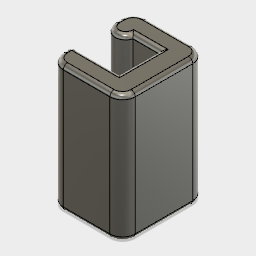
BedClamp v3 (Autodesk Fusion 360 design; units mm, degrees)
Autodesk Fusion 360 part; units mm, degrees
note: some values were not read from the file. Chosen so that the rebuilt part matches the saved one: which face or edge a step refers to. Set by a fixed rule: which sketch regions a step uses.
sketch "Sketch1" plane through (0, 0, 0) normal (0, 1, 0) x (1, 0, 0)
  line L0 (0, 0) -> (10, 0)
  line L1 (10, 0) -> (10, 8.8)
  line L2 (10, 8.8) -> (0, 8.8)
  line L3 (0, 0) -> (0, -5)
  line L4 (0, -5) -> (15, -5)
  line L5 (15, -5) -> (15, 0)
  line L6 (15, 0) -> (0, 0)
  line L7 (10, 0) -> (15, 0)
  line L8 (15, 0) -> (15, 13.8)
  line L9 (15, 13.8) -> (10, 13.8)
  line L10 (10, 13.8) -> (10, 0)
  line L11 (10, 13.8) -> (0, 13.8)
  line L12 (0, 13.8) -> (0, 8.8)
  line L13 (0, 8.8) -> (10, 8.8)
  line L14 (10, 8.8) -> (10, 13.8)
  line L15 (2.5, 7) -> (2.5, 9.5)
  circle A0 centre (2.5, 9.5) radius 2.5
  dimension "d1" = 8.8
  dimension "d2" = 13.8
  dimension "d4" = 2.5
  measures "d1" distance of L0.start L2.end
  measures "d2" distance of L0.end L9.end
  measures "d4" distance of L15.start L15.end
extrude "Extrude1" add sketch "Sketch1" along normal blind 30 contours L1 L6 L7 L8 L9 L10 L14 | L2 L10 L11 L12 L13 L14 A0 | L2 L13 L15 A0 | L2 L13 A0 | L2 L13 L15 A0 makes body 1
extrude "Extrude2" add 1 faces at (15, 10, -4.6) along direction (1, 0, 0) blind 10 on bodies 1 bodies 1
sketch "Sketch2" plane through (0, 0, 0) normal (0, 0, 1) x (1, 0, 0)
  line L0 (10, 0) -> (25, 0)
  line L1 (25, 0) -> (25, 30)
  line L2 (25, 30) -> (10, 30)
  line L3 (10, 30) -> (10, 0)
  line L4 (12, 15) -> (-113, 15)
  circle A0 centre (-113, 15) radius 125
  line L5 (17.5, 30) -> (17.5, 0)
  line L6 (17.5, 0) -> (0, 0)
  line L7 (0, 0) -> (0, 30)
  line L8 (0, 30) -> (17.5, 30)
  line L9 (0, 0) -> (0, 30)
  dimension "d9" = 125
  measures "d9" distance of L4.start L4.end
extrude "Extrude3" cut sketch "Sketch2" against normal blind 8.8 contours L0 L3 L4 A0 L6 | L2 L3 L4 A0 L8 bodies 1
sketch "Sketch3" plane through (0, 0, 0) normal (0, 0, 1) x (1, 0, 0)
  arc A0 (11.0967, 0) -> (11.0967, 30) centre (-113, 15) ccw
  line L0 (11.0967, 0) -> (25, 0)
  line L1 (25, 0) -> (25, 30)
  line L2 (25, 30) -> (11.0967, 30)
extrude "Extrude4" cut 1 faces at (25, 10, -4.6) along direction (-1, 0, 0) blind 8 on bodies 1 bodies 1
extrude "Extrude5" add sketch "Sketch2" along normal blind 5 contours L0 L2 A0 L5 L6 L8 | L0 L3 L4 A0 L6 | L3 L4 L6 L7 L9 | L2 L3 L4 A0 L8 | L3 L4 L7 L8 L9 bodies 1
extrude "Extrude6" cut 1 faces at (17.5, 20, 1.6667) along direction (-1, 0, 0) blind 0.5 on bodies 1 bodies 1
fillet "Fillet1" radius 1 1 edges at (0, 15, 0) on bodies 1
fillet "Fillet2" radius 3 4 edges at (17, 15, -13.8) (0, 15, -13.8) (0, 15, 5) (17, 15, 5) on bodies 1
fillet "Fillet3" radius 1 14 edges at (6.0484, 30, 0) (0.2929, 30, 0.2929) (0, 30, 1.5) (0.8787, 30, 4.1213) (8.5, 30, 5) (16.1213, 30, 4.1213) (17, 30, -4.4) (16.1213, 30, -12.9213) (8.5, 30, -13.8) (0.8787, 30, -12.9213) (0, 30, -10.15) (2.1464, 30, -7.0251) (7.9984, 30, -8.8) (11.0967, 30, -4.4) on bodies 1
fillet "Fillet4" radius 1 14 edges at (11.0967, 0, -4.4) (6.0484, 0, 0) (0.2929, 0, 0.2929) (0, 0, 1.5) (0.8787, 0, 4.1213) (8.5, 0, 5) (16.1213, 0, 4.1213) (17, 0, -4.4) (16.1213, 0, -12.9213) (8.5, 0, -13.8) (0.8787, 0, -12.9213) (0, 0, -10.15) (2.1464, 0, -7.0251) (7.9984, 0, -8.8) on bodies 1
ref_plane "WorkPlane1" through (8.5, 15, -3.8) normal (0, 0, -1) x (-1, 0, 0)
split "Split1" by plane through (8.5, 15, -3.8) normal (0, 0, -1) bodies 1 makes body 2 at (10.3333, 10.3333, -13.8)
move_body "Move1" bodies 2 to x (1, 0, 0) y (0, 1, 0) z (0, 0, 1) at (0, 0, -1.5)
extrude "Extrude7" add 1 faces at (15.3046, 16.546, -3.8) along direction (0, 0, -1) blind 0.75 on bodies 1 bodies 1
move_body "Move2" bodies 2 to x (1, 0, 0) y (0, 1, 0) z (0, 0, 1) at (0, 0, 0.75)
combine "Combine1" operation add target body 2 tool bodies 1
copy_body "Body->Comp1" bodies 2 removing the originals makes body 3 in component "BedClamp"
component "BedClamp" placed x (1, 0, 0) y (0, 1, 0) z (0, 0, 1) at (0, 0, 0)
equation "d2 = 8.800 mm + 5 mm"
